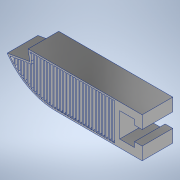
# Autodesk Inventor part: Finray_9_Kerbe_10deg
Saved by Autodesk Inventor 2022 (Build 260153000, 153)
## iProperties
Created: 2022-02-28
Part Number: Finray_9_Kerbe_10deg
Material: Generic
Document SubType Name: Modeling
Designer: richa
Density: 1 g/cm^3
Appearance: Aluminum - Flat
Author: richa
Autodesk Inventor part; units mm, degrees
ref_plane "YZ Plane" through (0, 0, 0) normal (1, 0, 0) x (0, 1, 0)
ref_plane "XZ Plane" through (0, 0, 0) normal (0, 1, 0) x (-1, 0, 0)
ref_plane "XY Plane" through (0, 0, 0) normal (0, 0, 1) x (1, 0, 0)
sketch "Sketch5" plane through (0, 0, 0) normal (0, 0, 1) x (1, 0, 0)
  line L0 (52.8, -15.6) -> (52.8, -10.6)
  line L1 (52.8, -10.6) -> (49.8, -10.6)
  line L2 (49.8, -10.6) -> (49.8, -12.6)
  line L3 (44, -12.6) -> (44, -3)
  line L4 (49.8, -3) -> (49.8, -5)
  line L5 (49.8, -5) -> (52.8, -5)
  line L6 (52.8, -5) -> (52.8, 0)
  line L7 (52.8, 0) -> (7.8, 0)
  line L8 (44, -3) -> (49.8, -3)
  line L9 (44, -12.6) -> (49.8, -12.6)
  line L10 (52.8, -15.6) -> (7.8, -15.6)
  line L11 (7.8, -15.6) -> (0, -15.6)
  line L12 (0, -15.6) -> (0, 0)
  line L13 (0, 0) -> (7.8, 0)
  point P0 (7.8, 0)
  dimension "d41" = 5.8
  dimension "d48" = 44
  dimension "d50" = 3
  dimension "d63" = 45
  dimension "d71" = 0
  dimension "d87" = 5.6
  dimension "d88" = 9.6
  dimension "d97" = 15.6
  constraints: 28 end point, 8 perpendicular, 4 collinear, 3 parallel, 2 horizontal, 1 vertical
  measures "d41" distance between parallel lines of L2 L3
  measures "d48" distance from line of L3 L12.end
  measures "d50" distance of L4.end L5.end
  measures "d63" distance of L0.start L10.end
  measures "d71" distance from line of L12.end L7
  measures "d87" distance from line of L0.end L5
  measures "d88" distance of L3.start L3.end
  measures "d97" distance of L11.end L12.end
extrude "Extrusion2" add sketch "Sketch5" along normal blind 12
sketch "Sketch8" plane through (0, 0, 0) normal (0, 0, -1) x (-1, 0, 0)
  line L0 (-8.1687, 0) -> (-8.8633, -3.9392)
  line L1 (-7.8, 0) -> (-1.143, 0) construction
  line L2 (0, -5.5021) -> (-8.8633, -3.9392)
  line L3 (-7.8, 0) -> (-8.1687, 0)
  line L4 (0, 0) -> (0, -15.6) projected
  line L5 (-52.8, 0) -> (0, 0) projected
  line L6 (-7.8, 0) -> (0, 0)
  line L7 (0, 0) -> (0, -5.5021)
  dimension "d80" = 100
  dimension "d95" = 4
  dimension "d96" = 9
  constraints: 12 end point, 2 collinear, 2 perpendicular, 1 horizontal, 1 point on line
  measures "d80" angle of L0 L1
  measures "d95" distance of L0.start L0.end
  measures "d96" distance of L2.start L0.end
extrude "Extrusion5" cut sketch "Sketch8" against normal through all
fillet "Fillet2" radius 23 1 edges at (0, -15.6, 6)
shell "Shell1" thickness 0.62 removed faces 1 at (23.9679, -7.5131, 12)
sketch "Sketch13" plane through (0, 0, 12) normal (0, 0, 1) x (1, 0, 0)
  line L0 (19.0404, -15.6) -> (52.8, -15.6) projected
  line L1 (42.0526, -15.6) -> (42.0526, 0)
  line L2 (52.8, 0) -> (8.1687, 0) projected
  line L3 (52.8, 0) -> (8.1687, 0) projected
  line L4 (52.8, -5) -> (52.8, 0) projected
  line L5 (49.8, -5) -> (52.8, -5) projected
  line L6 (49.8, -3) -> (49.8, -5) projected
  line L7 (44, -3) -> (49.8, -3) projected
  line L8 (44, -12.6) -> (44, -3) projected
  line L9 (49.8, -12.6) -> (44, -12.6) projected
  line L10 (49.8, -10.6) -> (49.8, -12.6) projected
  line L11 (52.8, -10.6) -> (49.8, -10.6) projected
  line L12 (52.8, -15.6) -> (52.8, -10.6) projected
  line L13 (42.0526, 0) -> (52.8, 0)
  line L14 (52.8, -5) -> (52.8, 0) projected
  line L15 (52.8, -5) -> (52.8, 0)
  line L16 (52.8, 0) -> (52.8, -5)
  line L17 (44, -12.6) -> (44, -3) projected
  line L18 (44, -3) -> (44, -12.6)
  line L19 (49.8, -12.6) -> (44, -12.6) projected
  line L20 (44, -12.6) -> (49.8, -12.6)
  line L21 (43.38, -13.22) -> (50.42, -13.22) projected
  line L22 (52.8, -10.6) -> (52.8, -15.6)
  line L23 (52.8, -15.6) -> (42.0526, -15.6)
  line L24 (44, -3) -> (49.8, -3) projected
  line L25 (44, -3) -> (49.8, -3)
  line L26 (49.8, -3) -> (49.8, -5)
  line L27 (49.8, -5) -> (52.8, -5)
  line L28 (52.8, -10.6) -> (49.8, -10.6)
  line L29 (49.8, -10.6) -> (49.8, -12.6)
  point P0 (0, 0)
  dimension "d102" = 10.7474
  constraints: 26 end point, 10 collinear, 2 point on line, 2 vertical, 1 parallel
  measures "d102" distance between parallel lines of L4 L1
extrude "Extrusion7" add sketch "Sketch13" against normal blind 12
sketch "Sketch14" plane through (8.9076, -0.62, 0.62) normal (0, 0, 1) x (1, 0, 0)
  line L0 (33.145, -14.36) -> (33.145, 0) projected
  line L1 (33.145, 0) -> (0, 0) projected
  line L2 (0.6739, -3.8221) -> (0, 0) projected
  line L3 (-7.835, -5.3225) -> (0.6739, -3.8221) projected
  arc A0 (-7.835, -5.3225) -> (10.1328, -14.36) centre (10.1328, 8.02) ccw projected
  line L4 (10.1328, -14.36) -> (33.145, -14.36) projected
  point P0 (-8.9076, 0.62)
extrude "Extrusion8" cut sketch "Sketch14" against normal blind 12
sketch "Sketch15" plane through (0, 0, 12) normal (0, 0, 1) x (1, 0, 0)
  line L0 (42.0526, -0.62) -> (8.9076, -0.62) construction
  line L1 (19.0404, -14.98) -> (42.0526, -14.98) projected
  line L2 (38.2426, -0.62) -> (38.6226, -0.62)
  line L3 (38.6226, -0.62) -> (38.6226, -14.98)
  line L4 (38.6226, -14.98) -> (38.2426, -14.98)
  line L5 (38.2426, -14.98) -> (38.2426, -0.62)
  line L6 (34.4326, -0.62) -> (34.8126, -0.62)
  line L7 (34.8126, -0.62) -> (34.8126, -14.98)
  line L8 (34.8126, -14.98) -> (34.4326, -14.98)
  line L9 (34.4326, -14.98) -> (34.4326, -0.62)
  line L10 (30.6226, -0.62) -> (31.0026, -0.62)
  line L11 (31.0026, -0.62) -> (31.0026, -14.98)
  line L12 (31.0026, -14.98) -> (30.6226, -14.98)
  line L13 (30.6226, -14.98) -> (30.6226, -0.62)
  line L14 (26.8126, -0.62) -> (27.1926, -0.62)
  line L15 (27.1926, -0.62) -> (27.1926, -14.98)
  line L16 (27.1926, -14.98) -> (26.8126, -14.98)
  line L17 (26.8126, -14.98) -> (26.8126, -0.62)
  line L18 (23.0026, -0.62) -> (23.3826, -0.62)
  line L19 (23.3826, -0.62) -> (23.3826, -14.98)
  line L20 (23.3826, -14.98) -> (23.0026, -14.98)
  line L21 (23.0026, -14.98) -> (23.0026, -0.62)
  line L22 (19.1926, -0.62) -> (19.5726, -0.62)
  line L23 (19.5726, -0.62) -> (19.5726, -14.98)
  line L24 (19.5726, -14.98) -> (19.1926, -14.98)
  line L25 (19.1926, -14.98) -> (19.1926, -0.62)
  line L26 (15.3826, -0.62) -> (15.7626, -0.62)
  line L27 (15.7626, -0.62) -> (15.7626, -14.98)
  line L28 (15.7626, -14.98) -> (15.3826, -14.98)
  line L29 (15.3826, -14.98) -> (15.3826, -0.62)
  line L30 (11.5726, -0.62) -> (11.9526, -0.62)
  line L31 (11.9526, -0.62) -> (11.9526, -14.4807)
  line L32 (11.5726, -14.3539) -> (11.5726, -0.62)
  arc A0 (1.0726, -5.9425) -> (19.0404, -14.98) centre (19.0404, 7.4) ccw projected
  line L33 (42.0526, -0.62) -> (42.0526, -14.98) projected
  line L34 (1.0726, -5.9425) -> (9.5815, -4.4421) projected
  arc A1 (0, -5.5021) -> (19.0404, -15.6) centre (19.0404, 7.4) ccw projected
  line L35 (4.3326, -5.3677) -> (3.9526, -5.3677)
  line L36 (3.9526, -5.3677) -> (3.9526, -9.9597)
  line L37 (3.9526, -9.9597) -> (4.3326, -9.9597)
  line L38 (4.3326, -9.9597) -> (4.3326, -5.3677)
  line L39 (8.1426, -4.6475) -> (7.7626, -4.6475)
  line L40 (7.7626, -4.6475) -> (7.7626, -12.5934)
  line L41 (7.7626, -12.5934) -> (8.1426, -12.5934)
  line L42 (8.1426, -12.5934) -> (8.1426, -4.6475)
  line L43 (42.0526, -14.98) -> (19.0404, -14.98) projected
  line L44 (40.7826, -14.98) -> (41.1626, -14.98)
  line L45 (41.1626, -14.98) -> (41.1626, -0.62)
  line L46 (41.1626, -0.62) -> (40.7826, -0.62)
  line L47 (40.7826, -0.62) -> (40.7826, -14.98)
  line L48 (8.9076, -0.62) -> (42.0526, -0.62) projected
  line L49 (36.9726, -0.62) -> (37.3526, -0.62)
  line L50 (37.3526, -0.62) -> (37.3526, -14.98)
  line L51 (37.3526, -14.98) -> (36.9726, -14.98)
  line L52 (36.9726, -14.98) -> (36.9726, -0.62)
  line L53 (33.1626, -0.62) -> (33.5426, -0.62)
  line L54 (33.5426, -0.62) -> (33.5426, -14.98)
  line L55 (33.5426, -14.98) -> (33.1626, -14.98)
  line L56 (33.1626, -14.98) -> (33.1626, -0.62)
  line L57 (29.3526, -0.62) -> (29.7326, -0.62)
  line L58 (29.7326, -0.62) -> (29.7326, -14.98)
  line L59 (29.7326, -14.98) -> (29.3526, -14.98)
  line L60 (29.3526, -14.98) -> (29.3526, -0.62)
  line L61 (25.5426, -0.62) -> (25.9226, -0.62)
  line L62 (25.9226, -0.62) -> (25.9226, -14.98)
  line L63 (25.9226, -14.98) -> (25.5426, -14.98)
  line L64 (25.5426, -14.98) -> (25.5426, -0.62)
  line L65 (21.7326, -0.62) -> (22.1126, -0.62)
  line L66 (22.1126, -0.62) -> (22.1126, -14.98)
  line L67 (22.1126, -14.98) -> (21.7326, -14.98)
  line L68 (21.7326, -14.98) -> (21.7326, -0.62)
  line L69 (17.9226, -0.62) -> (18.3026, -0.62)
  line L70 (18.3026, -0.62) -> (18.3026, -14.9678)
  line L71 (18.3026, -14.9678) -> (17.9226, -14.9678)
  line L72 (17.9226, -14.9678) -> (17.9226, -0.62)
  line L73 (14.1126, -0.62) -> (14.4926, -0.62)
  line L74 (14.4926, -0.62) -> (14.4926, -14.5131)
  line L75 (14.4926, -14.5131) -> (14.1126, -14.5131)
  line L76 (14.1126, -14.5131) -> (14.1126, -0.62)
  line L77 (10.3026, -0.62) -> (10.6826, -0.62)
  line L78 (10.6826, -0.62) -> (10.6826, -13.3608)
  line L79 (10.6826, -13.3608) -> (10.3026, -13.3608)
  line L80 (10.3026, -13.3608) -> (10.3026, -0.62)
  line L81 (3.0626, -5.5916) -> (2.6826, -5.5916)
  line L82 (2.6826, -5.5916) -> (2.6826, -8.8222)
  line L83 (2.6826, -8.8222) -> (3.0626, -8.8222)
  line L84 (3.0626, -8.8222) -> (3.0626, -5.5916)
  line L85 (6.8726, -4.9198) -> (6.4926, -4.9198)
  line L86 (6.4926, -4.9198) -> (6.4926, -11.8026)
  line L87 (6.8726, -11.8026) -> (6.8726, -4.9198)
  line L88 (39.5126, -0.62) -> (39.8926, -0.62)
  line L89 (39.8926, -0.62) -> (39.8926, -14.98)
  line L90 (39.8926, -14.98) -> (39.5126, -14.98)
  line L91 (39.5126, -14.98) -> (39.5126, -0.62)
  line L92 (35.7026, -0.62) -> (36.0826, -0.62)
  line L93 (36.0826, -0.62) -> (36.0826, -14.98)
  line L94 (36.0826, -14.98) -> (35.7026, -14.98)
  line L95 (35.7026, -14.98) -> (35.7026, -0.62)
  line L96 (31.8926, -0.62) -> (32.2726, -0.62)
  line L97 (32.2726, -0.62) -> (32.2726, -14.98)
  line L98 (32.2726, -14.98) -> (31.8926, -14.98)
  line L99 (31.8926, -14.98) -> (31.8926, -0.62)
  line L100 (28.0826, -0.62) -> (28.4626, -0.62)
  line L101 (28.4626, -0.62) -> (28.4626, -14.98)
  line L102 (28.4626, -14.98) -> (28.0826, -14.98)
  line L103 (28.0826, -14.98) -> (28.0826, -0.62)
  line L104 (24.2726, -0.62) -> (24.6526, -0.62)
  line L105 (24.6526, -0.62) -> (24.6526, -14.98)
  line L106 (24.6526, -14.98) -> (24.2726, -14.98)
  line L107 (24.2726, -14.98) -> (24.2726, -0.62)
  line L108 (20.4626, -0.62) -> (20.8426, -0.62)
  line L109 (20.8426, -0.62) -> (20.8426, -14.98)
  line L110 (20.8426, -14.98) -> (20.4626, -14.98)
  line L111 (20.4626, -14.98) -> (20.4626, -0.62)
  line L112 (16.6526, -0.62) -> (17.0326, -0.62)
  line L113 (17.0326, -0.62) -> (17.0326, -14.8898)
  line L114 (17.0326, -14.8898) -> (16.6526, -14.8898)
  line L115 (16.6526, -14.8898) -> (16.6526, -0.62)
  line L116 (12.8426, -0.62) -> (13.2226, -0.62)
  line L117 (13.2226, -0.62) -> (13.2226, -14.2106)
  line L118 (13.2226, -14.2106) -> (12.8426, -14.2106)
  line L119 (12.8426, -14.2106) -> (12.8426, -0.62)
  line L120 (5.6026, -5.1437) -> (5.2226, -5.1437)
  line L121 (5.2226, -5.1437) -> (5.2226, -10.6058)
  line L122 (5.2226, -10.6058) -> (5.6026, -10.6058)
  line L123 (5.6026, -10.6058) -> (5.6026, -5.1437)
  line L124 (9.4126, -0.62) -> (9.0326, -0.62)
  line L125 (9.0326, -0.62) -> (9.0326, -13.028)
  line L126 (9.0326, -13.028) -> (9.4126, -13.028)
  line L127 (9.4126, -13.028) -> (9.4126, -0.62)
  line L128 (6.4926, -11.8026) -> (6.8726, -11.8026)
  point P0 (0, 0)
  point P1 (11.5726, -13.6973)
  point P2 (11.9526, -13.828)
  point P3 (40.7826, -14.98)
  point P4 (41.1626, -14.98)
  point P5 (36.9726, -14.98)
  point P6 (37.3526, -14.98)
  point P7 (37.3526, -0.62)
  point P8 (33.1626, -0.62)
  point P9 (33.1626, -14.98)
  point P10 (33.5426, -14.98)
  point P11 (33.5426, -0.62)
  point P12 (29.3526, -0.62)
  point P13 (29.3526, -14.98)
  point P14 (29.7326, -14.98)
  point P15 (29.7326, -0.62)
  point P16 (25.5426, -0.62)
  point P17 (25.5426, -14.98)
  point P18 (25.9226, -14.98)
  point P19 (25.9226, -0.62)
  point P20 (21.7326, -0.62)
  point P21 (21.7326, -14.98)
  point P22 (22.1126, -14.98)
  point P23 (22.1126, -0.62)
  point P24 (18.3026, -0.62)
  point P25 (14.4926, -0.62)
  point P26 (10.6826, -0.62)
  dimension "d105" = 0.38
  dimension "d106" = 3.81
  dimension "d107" = 0.38
  dimension "d108" = 0.38
  dimension "d109" = 0.38
  dimension "d110" = 0.38
  dimension "d111" = 0.38
  dimension "d112" = 0.38
  dimension "d113" = 0.38
  dimension "d116" = 3.81
  dimension "d117" = 3.81
  dimension "d118" = 0.38
  dimension "d119" = 0.38
  dimension "d120" = 3.81
  dimension "d121" = 3.81
  dimension "d122" = 3.81
  dimension "d123" = 3.81
  dimension "d124" = 3.81
  dimension "d125" = 3.81
  dimension "d126" = 3.81
  dimension "d129" = 0.38
  dimension "d131" = 0.38
  dimension "d132" = 0.38
  dimension "d133" = 0.38
  dimension "d134" = 0.38
  dimension "d135" = 0.38
  dimension "d136" = 0.38
  dimension "d137" = 0.38
  dimension "d138" = 0.38
  dimension "d139" = 0.38
  dimension "d140" = 0.38
  dimension "d151" = 0.38
  dimension "d154" = 0.89
  dimension "d155" = 0.89
  dimension "d156" = 0.89
  dimension "d157" = 0.38
  dimension "d158" = 0.89
  dimension "d159" = 0.89
  dimension "d160" = 0.89
  dimension "d161" = 0.38
  dimension "d162" = 0.89
  dimension "d163" = 0.38
  dimension "d164" = 0.89
  dimension "d165" = 0.89
  dimension "d166" = 0.38
  dimension "d167" = 0.89
  dimension "d168" = 0.89
  dimension "d169" = 0.38
  dimension "d170" = 0.89
  dimension "d171" = 0.89
  dimension "d172" = 0.38
  dimension "d173" = 0.89
  dimension "d174" = 0.89
  dimension "d175" = 0.38
  dimension "d176" = 0.89
  dimension "d178" = 0.38
  dimension "d179" = 0.89
  dimension "d180" = 0.89
  dimension "d181" = 0.38
  dimension "d182" = 0.89
  dimension "d183" = 0.89
  dimension "d184" = 0.89
  constraints: 246 end point, 60 parallel, 32 perpendicular, 31 horizontal, 23 point on line, 8 point on circle, 29 other
  measures "d105" distance between parallel lines of L3 L5
  measures "d106" distance between parallel lines of L33 L5
  measures "d107" distance between parallel lines of L7 L9
  measures "d108" distance of L10.start L10.end
  measures "d109" distance of L14.start L14.end
  measures "d110" distance between parallel lines of L19 L21
  measures "d111" distance between parallel lines of L23 L25
  measures "d112" distance between parallel lines of L27 L29
  measures "d113" distance between parallel lines of L31 L32
  measures "d116" distance between parallel lines of L5 L9
  measures "d117" distance between parallel lines of L9 L13
  measures "d118" distance of L39.start L39.end
  measures "d119" distance of L35.start L35.end
  measures "d120" distance between parallel lines of L13 L17
  measures "d121" distance between parallel lines of L17 L21
  measures "d122" distance between parallel lines of L21 L25
  measures "d123" distance between parallel lines of L25 L29
  measures "d124" distance between parallel lines of L29 L32
  measures "d125" distance between parallel lines of L32 L40
  measures "d126" distance between parallel lines of L40 L36
  measures "d129" distance between parallel lines of L45 L47
  measures "d131" distance between parallel lines of L50 L52
  measures "d132" distance between parallel lines of L54 L56
  measures "d133" distance between parallel lines of L58 L60
  measures "d134" distance between parallel lines of L62 L64
  measures "d135" distance between parallel lines of L66 L68
  measures "d136" distance between parallel lines of L70 L72
  measures "d137" distance between parallel lines of L74 L76
  measures "d138" distance between parallel lines of L78 L80
  measures "d139" distance between parallel lines of L87 L86
  measures "d140" distance between parallel lines of L84 L82
  measures "d151" distance between parallel lines of L89 L91
  measures "d154" distance between parallel lines of L33 L45
  measures "d155" distance between parallel lines of L47 L89
  measures "d156" distance between parallel lines of L5 L50
  measures "d157" distance between parallel lines of L93 L95
  measures "d158" distance between parallel lines of L52 L93
  measures "d159" distance between parallel lines of L9 L54
  measures "d160" distance between parallel lines of L56 L97
  measures "d161" distance between parallel lines of L97 L99
  measures "d162" distance between parallel lines of L13 L58
  measures "d163" distance between parallel lines of L101 L103
  measures "d164" distance between parallel lines of L60 L101
  measures "d165" distance between parallel lines of L17 L62
  measures "d166" distance between parallel lines of L105 L107
  measures "d167" distance between parallel lines of L64 L105
  measures "d168" distance between parallel lines of L21 L66
  measures "d169" distance between parallel lines of L109 L111
  measures "d170" distance between parallel lines of L68 L109
  measures "d171" distance between parallel lines of L25 L70
  measures "d172" distance between parallel lines of L113 L115
  measures "d173" distance between parallel lines of L72 L113
  measures "d174" distance between parallel lines of L29 L74
  measures "d175" distance between parallel lines of L117 L119
  measures "d176" distance between parallel lines of L76 L117
  measures "d178" distance of L124.start L124.end
  measures "d179" distance between parallel lines of L80 L127
  measures "d180" distance between parallel lines of L40 L87
  measures "d181" distance between parallel lines of L123 L121
  measures "d182" distance between parallel lines of L86 L123
  measures "d183" distance between parallel lines of L36 L84
  measures "d184" distance between parallel lines of L32 L78
extrude "Extrusion9" add sketch "Sketch15" against normal blind 12 contours L25 L22 L23 L1 | L71 L72 A0 | A0 L72 L48 L70 | L111 L48 L109 L1 | L114 L115 A0 | A0 L115 L48 L113 | L68 L48 L66 L1 | A0 L29 L26 L27 | L27 L28 L29 A0 | L21 L18 L19 L1 | L75 L76 A0 | A0 L76 L48 L74 | L107 L48 L105 L1 | L118 L119 A0 | A0 L119 L48 L117 | L64 L48 L62 L1 | A0 L32 L30 L31 | L17 L14 L15 L1 | L79 L80 A0 | A0 L80 L48 L78 | L36 A0 L38 L37 | L103 L48 L101 L1 | L83 L82 A1 | A1 L82 A0 L84 L83 | L36 L34 L38 A0 | L127 L126 L125 A0 | A0 L125 L34 L127 | L127 L34 L125 L48 | A0 L82 L34 L84 | L36 L35 L34 | L60 L48 L58 L1 | L34 L82 L81 | L121 L34 L123 A0 | A0 L123 L122 L121 | L42 L41 L40 A0 | A0 L40 L34 L42 | L121 L120 L34 | L34 L40 L39 L42 | L13 L10 L11 L1 | L86 L34 L87 A0 | A0 L87 L128 L86 | L86 L85 L34 | L99 L48 L97 L1 | L56 L48 L54 L1 | L9 L6 L7 L1 | L95 L48 L93 L1 | L52 L48 L50 L1 | L5 L2 L3 L1 | L91 L48 L89 L1 | L47 L46 L45 L1
equation "\"l1\" = 8"
equation "\"d1\" = 0.38"
body "Solid2"
